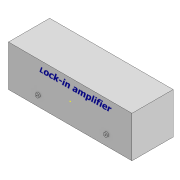
# Autodesk Inventor part: lock-in
Saved by Autodesk Inventor 2021 (Build 250183000, 183)
## iProperties
Created: 2022-02-10
Part Number: lock-in
Material: Типовые
Document SubType Name: Modeling
Designer: Тиннелла о Каллинике
Density: 1 g/cm^3
Appearance: По умолчанию
Author: Тиннелла о Каллинике
Autodesk Inventor part; units mm, degrees
ref_plane "YZ Plane" through (0, 0, 0) normal (1, 0, 0) x (0, 1, 0)
ref_plane "XZ Plane" through (0, 0, 0) normal (0, 1, 0) x (-1, 0, 0)
sketch "Эскиз1" plane through (0, 0, 0) normal (0, 0, 1) x (1, 0, 0)
  line L0 (-15, 5) -> (15, 5)
  line L1 (15, 5) -> (15, -5)
  line L2 (15, -5) -> (-15, -5)
  line L3 (-15, -5) -> (-15, 5)
  point P0 (0, 0)
  point P1 (0, 5)
  point P2 (15, 0)
  dimension "d0" = 30
  dimension "d1" = 10
  constraints: 8 end point, 2 midpoint, 2 parallel, 1 horizontal, 1 horizontal alignment, 1 perpendicular, 1 vertical alignment
  measures "d0" distance of L0.start L0.end
  measures "d1" distance of L0.end L1.end
extrude "Выдавливание1" add sketch "Эскиз1" against normal blind 10
sketch "Эскиз2" plane through (0, 0, 0) normal (0, 0, 1) x (1, 0, 0)
  line L0 (-7.5853, 4.0771) -> (10.7261, 4.0771) construction
  line L1 (10.7261, 4.0771) -> (10.7261, -0.5016) construction
  line L2 (10.7261, -0.5016) -> (-7.5853, -0.5016) construction
  line L3 (-7.5853, -0.5016) -> (-7.5853, 4.0771) construction
  point P0 (0, 0)
  constraints: 2 other
ref_plane "РабПлоскость1" through (0, 0, 0) normal (0, 0, 1) x (1, 0, 0)
sketch "Эскиз3" plane through (0, 0, 0) normal (0, 0, 1) x (1, 0, 0)
  circle A0 centre (-7.775, -2.4968) radius 0.5
  circle A1 centre (8.8496, -2.4968) radius 0.5
  point P0 (0, 0)
  dimension "d5" = 1
  dimension "d6" = 1
  constraints: 2 centre point
  measures "d5" diameter of A0
  measures "d6" diameter of A1
extrude "Выдавливание2" add sketch "Эскиз3" along normal blind 0.3
sketch "Эскиз4" plane through (0, 0, 0) normal (0, 0, 1) x (1, 0, 0)
  circle A0 centre (-7.775, -2.4968) radius 0.5 projected
  circle A1 centre (-7.775, -2.4968) radius 0.1
  circle A2 centre (8.8496, -2.4968) radius 0.5 projected
  circle A3 centre (8.8496, -2.4968) radius 0.1
  point P0 (0, 0)
  dimension "d9" = 0.2
  dimension "d10" = 0.2
  constraints: 2 centre point, 2 coincident
  measures "d9" diameter of A1
  measures "d10" diameter of A3
extrude "Выдавливание3" add sketch "Эскиз4" along normal blind 0.4 contours A1 | A3
